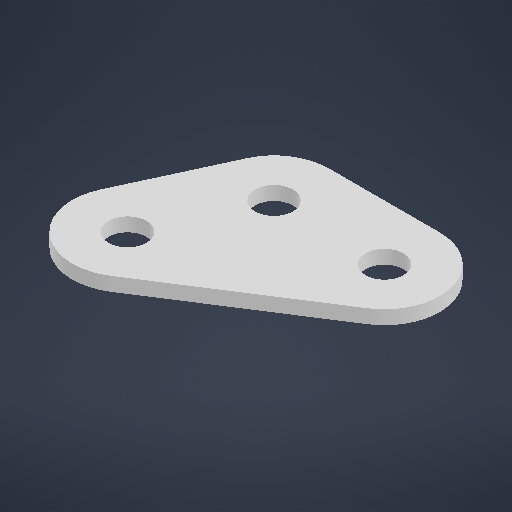
# Autodesk Inventor part: lbL-channelSupport
Saved by Autodesk Inventor 2025.2 (Build 292293000, 293)
## iProperties
Created: 2025-03-26
Part Number: lbL-channelSupport
Material: Generic
Document SubType Name: Modeling
Designer: Jahan
Density: 1 g/cm^3
Appearance: Default
Author: Jahan
Autodesk Inventor part; units mm, degrees
ref_plane "YZ Plane" through (0, 0, 0) normal (1, 0, 0) x (0, 1, 0)
ref_plane "XZ Plane" through (0, 0, 0) normal (0, 1, 0) x (-1, 0, 0)
ref_plane "XY Plane" through (0, 0, 0) normal (0, 0, 1) x (1, 0, 0)
sketch "Sketch1" plane through (0, 0, 0) normal (0, 1, 0) x (-1, 0, 0)
  circle A0 centre (-14.3247, -0.0006) radius 2.1844
  circle A1 centre (-1.6247, -0.0006) radius 2.1844
  circle A2 centre (3.6787, 11.5391) radius 2.1844
  circle A3 centre (3.6787, 11.5391) radius 6.35
  circle A4 centre (-1.6247, -0.0006) radius 6.35
  circle A5 centre (-14.3247, -0.0006) radius 6.35
  line L0 (0.252, 16.8851) -> (-17.7513, 5.3454)
  line L1 (-1.6231, -6.3506) -> (-14.3247, -6.3506)
  line L2 (4.1452, -2.6523) -> (9.4485, 8.8874)
  point P0 (0, 0)
  dimension "d0" = 12.7
  dimension "d1" = 12.7
  dimension "d2" = 12.7
  constraints: 6 centre point, 6 end point, 6 point on circle, 4 tangent, 3 coincident, 1 horizontal
  measures "d0" diameter of A3
  measures "d1" diameter of A4
  measures "d2" diameter of A5
extrude "Extrusion1" add sketch "Sketch1" along normal blind 1.5875
body "Solid1"
